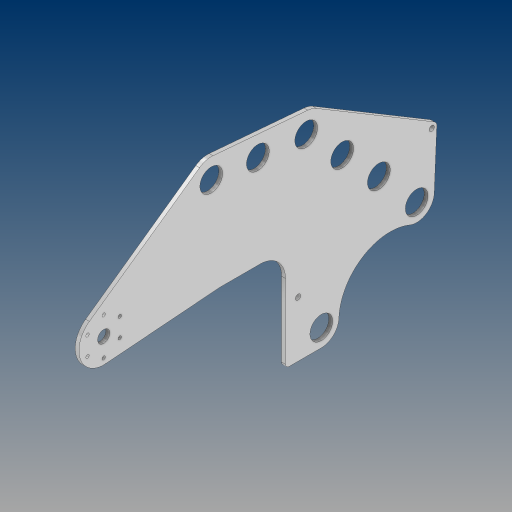
# Autodesk Inventor part: Intake Roller Plate
Saved by Autodesk Inventor 2024.3 (Build 283343000, 343)
## iProperties
Created: 2024-07-25
Part Number: Intake Roller Plate
Material: Aluminum 6061
Document SubType Name: Modeling
Designer: Kenji
Density: 2.7 g/cm^3
Appearance: Aluminum - Dark
Author: Kenji
Autodesk Inventor part; units mm, degrees
ref_plane "YZ Plane" through (0, 0, 0) normal (1, 0, 0) x (0, 1, 0)
ref_plane "XZ Plane" through (0, 0, 0) normal (0, 1, 0) x (-1, 0, 0)
ref_plane "XY Plane" through (0, 0, 0) normal (0, 0, 1) x (1, 0, 0)
sketch "Sketch1" plane through (0, 0, 0) normal (1, 0, 0) x (0, 1, 0)
  line L0 (127, 0) -> (127, -31.75) construction
  line L1 (95.25, -63.5) -> (31.75, -63.5) construction
  line L2 (0, -31.75) -> (0, 0) construction
  arc A0 (95.25, -63.5) -> (127, -31.75) centre (95.25, -31.75) ccw construction
  arc A1 (0, -31.75) -> (31.75, -63.5) centre (31.75, -31.75) ccw construction
  line L3 (0, 0) -> (0, 19.05) construction
  line L4 (0, 19.05) -> (-12.7, 19.05) construction
  line L5 (82.55, 19.05) -> (82.55, 292.1) construction
  circle A2 centre (82.55, 292.1) radius 25.4 construction
  circle A3 centre (82.55, 292.1) radius 31.75 construction
  circle A4 centre (231.775, 292.1) radius 25.4 construction
  circle A5 centre (231.775, 292.1) radius 31.75 construction
  line L6 (-12.7, 19.05) -> (82.55, 19.05) construction
  line L7 (127, 0) -> (0, 0) construction
  line L8 (-12.7, 19.05) -> (-12.7, -285.75) construction
  circle A6 centre (38.1, -179.2153) radius 50.8 construction
  circle A7 centre (95.7575, -229.0356) radius 25.4 construction
  circle A8 centre (95.7575, -229.0356) radius 14.2875
  circle A9 centre (147.9035, -181.2855) radius 25.4 construction
  circle A10 centre (147.9035, -181.2855) radius 14.2875
  circle A11 centre (239.6405, -89.6692) radius 22.225 construction
  circle A12 centre (239.6405, -89.6692) radius 25.4 construction
  circle A13 centre (239.6405, -89.6692) radius 14.2875
  line L9 (82.55, 19.05) -> (127, 19.05) construction
  line L10 (127, 19.05) -> (127, 0) construction
  circle A14 centre (147.9035, -181.2855) radius 22.225 construction
  circle A15 centre (95.7575, -229.0356) radius 22.225 construction
  circle A16 centre (19.05, -108.7189) radius 25.4 construction
  circle A17 centre (19.05, -108.7189) radius 22.225 construction
  line L11 (19.05, -83.3189) -> (19.05, -63.5) construction
  circle A18 centre (194.4203, -135.0384) radius 25.4 construction
  circle A19 centre (194.4203, -135.0384) radius 22.225 construction
  circle A20 centre (194.4203, -135.0384) radius 14.2875
  line L12 (-6.35, -108.7189) -> (-12.7, -108.7189) construction
  circle A21 centre (66.911, -79.375) radius 6.477 construction
  circle A22 centre (19.05, -108.7189) radius 14.2875
  circle A23 centre (66.911, -79.375) radius 3.2512
  circle A24 centre (79.9729, -154.4883) radius 50.8 construction
  circle A25 centre (126.5277, -108.1451) radius 50.8 construction
  circle A26 centre (104.7382, -122.3838) radius 50.8 construction
  circle A27 centre (171.9706, -62.2205) radius 50.8 construction
  circle A28 centre (166.8773, -248.0094) radius 3.2512
  circle A29 centre (244.7666, -28.6705) radius 14.2875
  circle A30 centre (244.7666, -28.6705) radius 22.225 construction
  line L13 (172.3896, -251.3125) -> (261.4282, -102.7251)
  line L14 (194.4203, -135.0384) -> (147.9035, -181.2855) construction
  line L15 (147.9035, -181.2855) -> (95.7575, -229.0356) construction
  line L16 (82.55, 19.05) -> (31.75, 19.05) construction
  line L17 (31.75, 19.05) -> (31.75, 292.1) construction
  line L18 (31.75, 292.1) -> (82.55, 292.1) construction
  arc A31 (261.4282, -102.7251) -> (264.9513, -91.7962) centre (239.6405, -89.6692) ccw
  circle A32 centre (177.8, 17.333) radius 50.8 construction
  circle A33 centre (249.7038, 30.0805) radius 14.2875
  circle A34 centre (249.7038, 30.0805) radius 22.225 construction
  circle A35 centre (244.7666, -28.6705) radius 7.62 construction
  circle A36 centre (249.7038, 30.0805) radius 25.4 construction
  line L19 (264.9513, -91.7962) -> (275.0146, 27.9535)
  line L20 (-12.7, -285.75) -> (571.5, -285.75) construction
  line L21 (571.5, -285.75) -> (571.5, 292.1) construction
  line L22 (31.75, 292.1) -> (571.5, 292.1) construction
  line L23 (127, 19.05) -> (571.5, 19.05) construction
  circle A37 centre (146.5717, 165.8007) radius 7.62
  circle A38 centre (146.5717, 165.8007) radius 23.495 construction
  circle A39 centre (170.0667, 165.8007) radius 2.0828
  circle A40 centre (146.5717, 165.8007) radius 27.94 construction
  line L24 (115.5542, 163.3402) -> (126.985, 19.2385)
  arc A41 (275.0146, 27.9535) -> (270.4313, 44.7615) centre (249.7038, 30.0805) ccw
  circle A42 centre (146.5717, 165.8007) radius 31.115 construction
  line L25 (270.4313, 44.7615) -> (171.9629, 183.7849)
  arc A43 (171.9629, 183.7849) -> (115.5542, 163.3402) centre (146.5717, 165.8007) ccw
  circle A44 centre (158.3192, 186.1479) radius 2.0828
  circle A45 centre (134.8242, 186.1479) radius 2.0828
  circle A46 centre (123.0767, 165.8007) radius 2.0828
  circle A47 centre (134.8242, 145.4534) radius 2.0828
  circle A48 centre (158.3192, 145.4534) radius 2.0828
  line L26 (-12.7, -63.5) -> (368.3, -63.5) construction
  arc A49 (75.2239, -220.5312) -> (94.7731, -251.2387) centre (95.7575, -229.0356) ccw
  circle A50 centre (166.8773, -248.0094) radius 6.4262 construction
  line L27 (166.8773, -254.4356) -> (94.7731, -251.2387)
  arc A51 (166.8773, -254.4356) -> (172.3896, -251.3125) centre (166.8773, -248.0094) ccw
  line L28 (368.3, -63.5) -> (368.3, -285.75) construction
  line L29 (2.3994, -123.4399) -> (81.0365, -212.3849) construction
  circle A52 centre (66.911, -79.375) radius 6.35 construction
  line L30 (127, 18.8609) -> (127, -31.75)
  line L31 (95.25, -63.5) -> (1.6002, -63.5)
  line L32 (-3.175, -68.2752) -> (-3.175, -108.7189)
  arc A53 (1.6002, -63.5) -> (-3.175, -68.2752) centre (1.6002, -68.2752) ccw
  arc A54 (95.25, -63.5) -> (127, -31.75) centre (95.25, -31.75) ccw
  arc A55 (127, 18.8609) -> (126.985, 19.2385) centre (122.2248, 18.8609) ccw
  arc A56 (-3.175, -108.7189) -> (18.0948, -130.9234) centre (19.05, -108.7189) ccw
  line L33 (249.7038, 30.0805) -> (239.6405, -89.6692) construction
  circle A57 centre (244.7666, -28.6705) radius 25.4 construction
  arc A58 (75.2239, -220.5312) -> (18.0948, -130.9234) centre (15.3074, -195.7156) ccw
  point P0 (-12.7, -179.2153)
  point P1 (173.3035, -181.2855)
  point P2 (104.775, 19.05)
  point P3 (173.3035, -248.0094)
  point P4 (95.7575, -254.4356)
  point P5 (127, -63.5)
  point P6 (-3.175, -63.5)
  dimension "d58" = 101.6
  dimension "d284" = 46.99
  dimension "d2" = 31.75
  dimension "d3" = 19.05
  dimension "d4" = 12.7
  dimension "d7" = 273.05
  dimension "d8" = 50.8
  dimension "d9" = 6.35
  dimension "d10" = 50.8
  dimension "d11" = 6.35
  dimension "d12" = 149.225
  dimension "d14" = 127
  dimension "d16" = 304.8
  dimension "d175" = 31.75
  dimension "d180" = 50.8
  dimension "d181" = 3.175
  dimension "d187" = 31.75
  dimension "d189" = 6.35
  dimension "d191" = 12.954
  dimension "d192" = 28.575
  dimension "d201" = 6.5024
  dimension "d207" = 101.6
  dimension "d208" = 101.6
  dimension "d210" = 130.175
  dimension "d214" = 15.875
  dimension "d216" = 101.6
  dimension "d218" = 6.5024
  dimension "d219" = 108.4575
  dimension "d220" = 143.1895
  dimension "d221" = 155.574
  dimension "d222" = 70.7056
  dimension "d236" = 50.8
  dimension "d237" = 44.45
  dimension "d261" = 166.37
  dimension "d267" = 15.24
  dimension "d271" = 584.2
  dimension "d283" = 15.24
  dimension "d285" = 4.1656
  dimension "d290" = 55.88
  dimension "d292" = 3.175
  dimension "d313" = 146.7507
  dimension "d318" = 114.8217
  dimension "d321" = 360
  dimension "d323" = 381
  dimension "d328" = 3.175
  dimension "d336" = 12.7
  dimension "d339" = 4.7752
  dimension "d340" = 31.75
  dimension "d341" = 4.7752
  dimension "d342" = 19.8189
  dimension "d343" = 33.0042
  dimension "d344" = 64.0217
  dimension "d360" = 120.1718
  dimension "d361" = 61.2137
  constraints: 69 end point, 54 centre point, 39 point on circle, 31 tangent, 21 point on line, 17 equal radius, 15 coincident, 11 perpendicular, 9 horizontal alignment, 8 concentric, 4 horizontal, 4 vertical, 4 vertical alignment, 3 parallel, 1 collinear, 1 midpoint, 35 other
  measures "d2" radius of A0
  measures "d3" distance of L2.end L3.end
  measures "d4" distance of L3.end L4.end
  measures "d7" distance of L5.start L5.end
  measures "d8" diameter of A2
  measures "d9" radial gap between concentric circles of A2 A3
  measures "d10" diameter of A4
  measures "d11" radial gap between concentric circles of A4 A5
  measures "d12" distance of L18.end A4.centre
  measures "d14" distance of L0.start L2.end
  measures "d16" distance of L4.end L8.end
  measures "d175" radius of A1
  measures "d180" diameter of A16
  measures "d181" radial gap between concentric circles of A16 A17
  measures "d187" distance of L0.start L0.end
  measures "d189" distance of L12.start L12.end
  measures "d191" diameter of A21
  measures "d192" diameter of A22
  measures "d201" diameter of A23
  measures "d207" diameter of A24
  measures "d208" diameter of A25
  measures "d210" distance of A21.centre A14.centre
  measures "d214" distance from line of L1 A21.centre
  measures "d216" diameter of A27
  measures "d218" diameter of A28
  measures "d219" distance from line of L8 point (95.757, -229.036)
  measures "d220" distance of A0.centre A18.centre
  measures "d221" distance of A0.centre A11.centre
  measures "d222" distance of point (95.757, -229.036) A14.centre
  measures "d236" distance of L5.start L16.end
  measures "d237" distance of L4.end L16.end
  measures "d261" distance of A0.centre A34.centre
  measures "d267" diameter of A35
  measures "d271" distance of L8.end L20.end
  measures "d283" diameter of A37
  measures "d285" diameter of A39
  measures "d290" diameter of A40
  measures "d313" distance from line of L9 point (146.572, 165.801)
  measures "d318" distance from line of L17 point (146.572, 165.801)
  measures "d323" distance of L26.start L26.end
  measures "d328" radial gap between concentric circles of A28 A50
  measures "d336" diameter of A52
  measures "d339" radius of A53
  measures "d340" radius of A54
  measures "d341" radius of A55
  measures "d342" distance of L11.end L11.start
  measures "d343" distance from line of L5 L24.start
  measures "d344" distance from line of L5 A40.centre
  measures "d360" distance of L33.start L33.end
  measures "d361" distance of A30.centre A11.centre
extrude "Extrusion7" add sketch "Sketch1" along normal blind 4.7625
body "Solid6"
